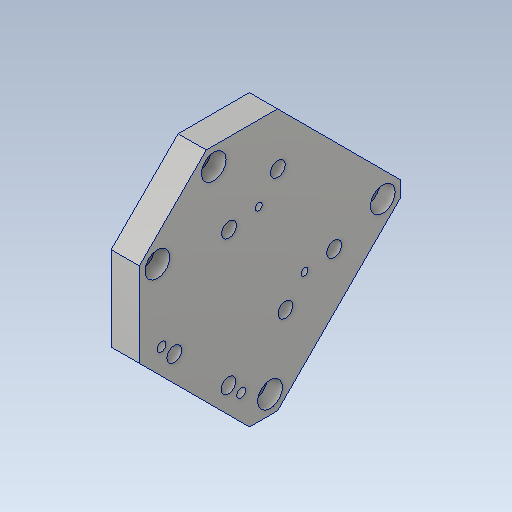
# Autodesk Inventor part: FAB-OX0003
Saved by Autodesk Inventor 2020 (Build 240168000, 168)
## iProperties
Created: 2016-12-07
Part Number: FAB-OX0003
Material: Aluminum 6061
Document SubType Name: Modeling
Designer: map
Density: 2.7 g/cm^3
Appearance: Aluminum - Flat
Mass: 272.856 g
Surface Area: 258.229 cm^2
Volume: 101.058 cm^3
Description: Lower wedge baseplate
d6: 8.000 mm
d8: 135.00 deg
d10: 135.00 deg
d11: 135.00 deg
d13: 8.000 mm
d14: 8.000 mm
d15: 8.000 mm
d18: 8.000 mm
d19: 8.000 mm
d20: 12.500 mm
d21: 0.00 deg
d43: 6.600 mm
d45: 11.000 mm
d46: 6.800 mm
d50: 6.600 mm
d52: 11.000 mm
d53: 6.800 mm
d64: 0.125 in
d69: 3.500 mm
d70: 118.00 deg
d71: 4.000 mm
d76: 8.000 mm
d77: 118.00 deg
d78: 2.500 mm
d79: 4.000 mm
d80: 4.000 mm
d88: 0.00 deg
d96: 6.000 mm
d97: 16.000 mm
d99: 8.000 mm
d103: 11.800 mm
d104: 118.00 deg
border: 8.000 mm
Author: map
Revision Number: 02
Autodesk Inventor part; units mm, degrees
ref_plane "YZ Plane" through (0, 0, 0) normal (1, 0, 0) x (0, 1, 0)
ref_plane "XZ Plane" through (0, 0, 0) normal (0, 1, 0) x (-1, 0, 0)
ref_plane "XY Plane" through (0, 0, 0) normal (0, 0, 1) x (1, 0, 0)
sketch "Sketch4" plane through (0, 0, 0) normal (1, 0, 0) x (0, 1, 0)
  line L0 (-56.119, -133.197) -> (-1.4327, -78.5108)
  line L1 (-68.5481, -17.197) -> (-117.4327, -66.0816)
  line L2 (-117.4327, -66.0816) -> (-117.4327, -78.5108)
  line L3 (-72.7358, -32.6985) -> (-96.7775, -56.7401) construction
  line L4 (-68.5481, -17.197) -> (-31.119, -17.197)
  line L5 (-1.4327, -78.5108) -> (-1.4327, -46.8833)
  line L6 (-1.4327, -46.8833) -> (-31.119, -17.197)
  line L7 (-56.119, -133.197) -> (-62.7464, -133.197)
  line L8 (-117.4327, -78.5108) -> (-62.7464, -133.197)
  circle A0 centre (-72.7358, -32.6985) radius 2.4585 projected
  circle A1 centre (-96.7775, -56.7401) radius 2.4585 projected
  point P0 (0, 0)
  point P1 (-59.4327, -125.197)
  point P2 (-34.4327, -25.197)
  point P3 (-9.4327, -50.197)
  point P4 (-109.4327, -75.197)
  dimension "d6" = 8
  dimension "d8" = 135
  dimension "d10" = 135
  dimension "d11" = 135
  dimension "d13" = 8
  dimension "d14" = 8
  dimension "d15" = 8
  dimension "d18" = 8
  dimension "d19" = 8
  dimension "d105" = 135
  dimension "d106" = 8
  dimension "d107" = 8
  constraints: 18 end point, 2 coincident, 2 horizontal, 1 vertical
  measures "d6" distance between parallel lines of L1 L3
  measures "d8" angle of L6 L4
  measures "d10" angle of L2 L1
  measures "d11" angle of L8 L2
  measures "d13" distance from line of L5 point (-9.433, -50.197)
  measures "d14" distance from line of point (-9.433, -50.197) L6
  measures "d15" distance from line of L4 point (-34.433, -25.197)
  measures "d18" distance from line of point (-59.433, -125.197) L7
  measures "d19" distance from line of point (-59.433, -125.197) L0
  measures "d105" angle of L0 L5
  measures "d106" distance from line of L8 point (-109.433, -75.197)
  measures "d107" distance from line of L2 point (-109.433, -75.197)
extrude "Extrusion2" add sketch "Sketch4" along normal blind 12.5 contours L7 L8 L2 L1 L4 L6 L5 L0 | A0 | A1
sketch "Sketch9" plane through (0, 0, 0) normal (-1, 0, 0) x (0, 0, 1)
  circle A0 centre (-78.6225, -24.5414) radius 2.5 projected
  circle A1 centre (-56.9775, -37.0382) radius 2.5 projected
  circle A2 centre (-103.6161, -67.8315) radius 2.5 projected
  circle A3 centre (-81.9711, -80.3283) radius 2.5 projected
  circle A4 centre (-32.6985, -72.7358) radius 2.4585 projected
  circle A5 centre (-56.7401, -96.7775) radius 2.4585 projected
hole "M6ClearanceToPayload" at (0, -24.5414, -78.6225) at (0, -37.0382, -56.9775) at (0, -80.3283, -81.9711) at (0, -67.8315, -103.6161) at (0, -96.7775, -56.7401) at (0, -72.7358, -32.6985) direction (1, 0, 0) diameter 6.6 end through all counterbore diameter 11 counterbore depth 6.8 clearance for "Socket Head Cap Screw ISO 4762" size "M6" standard "ISO"
sketch "Sketch11" plane through (12.5, 0, 0) normal (1, 0, 0) x (0, 0, -1)
  circle A0 centre (70.1368, -34.8372) radius 1.6002 projected
  circle A1 centre (90.4568, -70.0325) radius 1.6002 projected
hole "1/8\" dowel holes" at (12.5, -34.8372, -70.1368) at (12.5, -70.0325, -90.4568) direction (-1, 0, 0) diameter 3.175 depth 3.5 tip angle 118
sketch "Sketch12" plane through (12.5, 0, 0) normal (1, 0, 0) x (0, 0, -1)
  line L0 (63.8112, -101.0201) -> (60.9827, -103.8485)
  circle A0 centre (27.0416, -67.079) radius 2 projected
  line L1 (61.6898, -104.5556) -> (60.2756, -103.1414) projected
  line L2 (63.104, -100.313) -> (64.5183, -101.7272) projected
  point P0 (27.0416, -67.079)
  point P1 (62.3969, -102.4343)
  point P2 (27.0416, -67.079)
  constraints: 3 midpoint, 2 end point, 1 coincident
hole "4P6 dowel holes" at (12.5, -67.079, -27.0416) at (12.5, -102.4343, -62.3969) direction (-1, 0, 0) diameter 4 depth 8 tip angle 118
sketch "Sketch8" plane through (12.5, 0, 0) normal (1, 0, 0) x (0, 0, -1)
  point P0 (25.197, -34.4327)
  point P1 (50.197, -9.4327)
  point P2 (125.197, -59.4327)
  point P3 (75.197, -109.4327)
hole "M6ClearanceToSubstrate" at (12.5, -34.4327, -25.197) at (12.5, -9.4327, -50.197) at (12.5, -59.4327, -125.197) at (12.5, -109.4327, -75.197) direction (-1, 0, 0) diameter 6.6 end through all counterbore diameter 11 counterbore depth 6.8 clearance for "Socket Head Cap Screw ISO 4762" size "M6" standard "ISO"
sketch "Sketch13" plane through (0, 0, 0) normal (-1, 0, 0) x (0, 0, 1)
  circle A0 centre (-50.197, -9.4327) radius 3.3 projected
  circle A1 centre (-25.197, -34.4327) radius 3.3 projected
  line L0 (-50.197, -9.4327) -> (-25.197, -34.4327) construction
  circle A2 centre (-125.197, -59.4327) radius 3.3 projected
  circle A3 centre (-75.197, -109.4327) radius 3.3 projected
  line L1 (-125.197, -59.4327) -> (-75.197, -109.4327) construction
  line L2 (-37.697, -21.9327) -> (-100.197, -84.4327)
  line L3 (-35.9293, -20.1649) -> (-39.4648, -23.7004) construction
  line L4 (-37.3435, -18.7507) -> (-40.879, -22.2862)
  line L5 (-38.0506, -25.1147) -> (-34.5151, -21.5791)
  arc A4 (-34.5151, -21.5791) -> (-37.3435, -18.7507) centre (-35.9293, -20.1649) ccw
  arc A5 (-40.879, -22.2862) -> (-38.0506, -25.1147) centre (-39.4648, -23.7004) ccw
  dimension "d78" = 2.5
  dimension "d79" = 4
  constraints: 14 end point, 4 point on circle, 4 tangent, 3 coincident, 3 midpoint, 2 centre point, 1 parallel, 1 point on line
  measures "d78" distance of L2.start L3.end
  measures "d79" diameter of A5
hole "4H7 location holes" at (0, -20.1649, -35.9293) at (0, -23.7004, -39.4648) at (0, -84.4327, -100.197) direction (1, 0, 0) diameter 4 depth 8
extrude "Extrusion3" cut sketch "Sketch13" against normal blind 8 contours A4 L5 A5 L4
sketch "Sketch16" plane through (0, -117.4327, -66.0816) normal (0, -0.7071, 0.7071) x (1, 0, 0)
  line L0 (0, 21.2109) -> (12.5, 21.2109) construction
  line L1 (0, 55.2109) -> (11.8351, 55.2109) construction
  line L2 (6.5, 21.2109) -> (6.5, 55.2109) construction
  line L3 (12.5, 69.1332) -> (12.5, 0) construction
  line L4 (1.6198, 38.2109) -> (11.3802, 38.2109)
  line L5 (6.8, 49.7109) -> (6.8, 60.7109) projected
  line L6 (6.8, 15.7109) -> (6.8, 26.7109) projected
  line L7 (0, 49.7109) -> (0, 60.7109) projected
  line L8 (0, 15.7109) -> (0, 26.7109) projected
  point P0 (6.5, 38.2109)
  point P1 (6.5, 30.2109)
  point P2 (6.5, 46.2109)
  point P3 (6.8, 21.2109)
  dimension "d96" = 6
  dimension "d97" = 16
  constraints: 8 end point, 5 midpoint, 5 point on line, 2 horizontal, 1 perpendicular, 1 symmetric about line, 1 other
  measures "d96" distance between parallel lines of L2 L3
  measures "d97" distance of point (6.5, 46.211) point (6.5, 30.211)
hole "Hole11" at (6.5, -96.0704, -44.7193) at (6.5, -84.7567, -33.4056) direction (0, 0.7071, -0.7071) diameter 3.242 depth 11.8 tip angle 118 thread size "M4x0.7" class "6H" standard "ISO Metric profile"
equation "\"d6\" = border"
equation "\"d10\" = d8"
equation "\"d11\" = d8"
equation "\"d13\" = d15"
equation "\"d14\" = d15"
equation "\"d15\" = border"
equation "\"d18\" = d15"
equation "\"d19\" = d15"
equation "\"d105\" = d10"
equation "\"d106\" = d18"
equation "\"d107\" = d18"
equation "\"d64\" = thorlabsPinDiameter"
equation "\"border\" = 8"
equation "\"thorlabsPinDiameter\" = 3.175"
body "Solid2"
